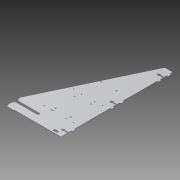
# Autodesk Inventor part: side_frame
Saved by Autodesk Inventor 2013 (Build 170138000, 138)
## iProperties
Created: 2013-11-17
Part Number: side_frame
Material: Generic
Document SubType Name: Modeling
Designer: Masta
Density: 1 g/cm^3
Author: Masta
Autodesk Inventor part; units mm, degrees
ref_plane "YZ Plane" through (0, 0, 0) normal (1, 0, 0) x (0, 1, 0)
ref_plane "XZ Plane" through (0, 0, 0) normal (0, 1, 0) x (-1, 0, 0)
ref_plane "XY Plane" through (0, 0, 0) normal (0, 0, 1) x (1, 0, 0)
sketch "Sketch1" plane through (0, 0, 0) normal (0, 0, 1) x (1, 0, 0)
  line L0 (255.7808, 350.0828) -> (255.7808, 358.8828)
  line L1 (251.6808, 67.29) -> (255.7808, 67.29)
  line L2 (255.7808, 67.29) -> (255.7808, 76.09)
  line L3 (255.7808, 76.09) -> (251.6808, 76.09)
  line L4 (251.6808, 76.09) -> (251.6808, 194.9901)
  line L5 (251.6808, 32.5401) -> (100.8808, 32.5401)
  line L6 (231.7439, 44.5401) -> (223.7479, 44.5401)
  line L7 (230.5808, 213.3401) -> (234.5808, 213.3401)
  line L8 (234.5808, 211.5401) -> (239.6808, 211.5401)
  line L9 (251.6808, 57.7345) -> (239.6808, 57.7345)
  line L10 (239.6808, 57.7345) -> (239.6808, 59.5345)
  line L11 (230.5808, 53.3345) -> (234.5808, 53.3345)
  line L12 (234.5808, 51.5345) -> (239.6808, 51.5345)
  line L13 (239.6808, 59.5345) -> (234.5808, 59.5345)
  line L14 (234.5808, 53.3345) -> (234.5808, 51.5345)
  line L15 (239.6808, 53.3345) -> (251.6808, 53.3345)
  line L16 (239.6808, 51.5345) -> (239.6808, 53.3345)
  line L17 (251.6808, 57.7345) -> (251.6808, 67.29)
  line L18 (251.6808, 217.7401) -> (239.6808, 217.7401)
  line L19 (255.7808, 236.0901) -> (251.6808, 236.0901)
  line L20 (251.6808, 236.0901) -> (251.6808, 350.0828)
  line L21 (255.7808, 203.7901) -> (251.6808, 203.7901)
  line L22 (251.6808, 194.9901) -> (255.7808, 194.9901)
  line L23 (255.7808, 194.9901) -> (255.7808, 203.7901)
  line L24 (251.6808, 227.2901) -> (251.6808, 217.7401)
  line L25 (251.6808, 213.3401) -> (251.6808, 203.7901)
  line L26 (251.6808, 382.3828) -> (255.7808, 382.3828)
  line L27 (255.7808, 382.3828) -> (255.7808, 391.1828)
  line L28 (255.7808, 391.1828) -> (251.6808, 391.1828)
  line L29 (251.6808, 391.1828) -> (251.6808, 400.5401)
  line L30 (255.7808, 358.8828) -> (251.6808, 358.8828)
  line L31 (251.6808, 350.0828) -> (255.7808, 350.0828)
  line L32 (73.8808, 35.5401) -> (73.8808, 51.1401)
  line L33 (239.6808, 211.5401) -> (239.6808, 213.3401)
  line L34 (230.5808, 217.7401) -> (230.5808, 213.3401)
  line L35 (73.8808, 77.5401) -> (226.2808, 400.5401)
  line L36 (234.5808, 217.7401) -> (230.5808, 217.7401)
  line L37 (234.5808, 217.7401) -> (234.5808, 219.5401)
  line L38 (251.6808, 400.5401) -> (226.2808, 400.5401)
  line L39 (239.6808, 213.3401) -> (251.6808, 213.3401)
  line L40 (231.7439, 36.5395) -> (223.7482, 36.5395)
  line L41 (239.6808, 219.5401) -> (234.5808, 219.5401)
  line L42 (98.8808, 30.5401) -> (78.8808, 30.5401)
  line L43 (234.5808, 213.3401) -> (234.5808, 211.5401)
  line L44 (230.5808, 372.825) -> (230.5808, 368.425)
  line L45 (234.5808, 372.825) -> (230.5808, 372.825)
  line L46 (234.5808, 372.825) -> (234.5808, 374.625)
  line L47 (251.6808, 372.825) -> (239.6808, 372.825)
  line L48 (230.5808, 368.425) -> (234.5808, 368.425)
  line L49 (239.6808, 368.425) -> (251.6808, 368.425)
  line L50 (234.5808, 366.625) -> (239.6808, 366.625)
  line L51 (239.6808, 374.625) -> (234.5808, 374.625)
  line L52 (234.5808, 368.425) -> (234.5808, 366.625)
  line L53 (251.6808, 372.825) -> (251.6808, 382.3828)
  line L54 (251.6808, 368.425) -> (251.6808, 358.8828)
  line L55 (230.5808, 57.7345) -> (230.5808, 53.3345)
  line L56 (234.5808, 57.7345) -> (230.5808, 57.7345)
  line L57 (234.5808, 57.7345) -> (234.5808, 59.5345)
  line L58 (239.6808, 366.625) -> (239.6808, 368.425)
  line L59 (239.6808, 372.825) -> (239.6808, 374.625)
  line L60 (78.8808, 56.1401) -> (148.8808, 56.1401)
  line L61 (78.8808, 56.1401) -> (73.8808, 51.1401)
  line L62 (78.8808, 64.9401) -> (148.8808, 64.9401)
  line L63 (73.8808, 69.9401) -> (73.8808, 77.5401)
  line L64 (78.8808, 64.9401) -> (73.8808, 69.9401)
  line L65 (251.6808, 227.2901) -> (255.7808, 227.2901)
  line L66 (255.7808, 227.2901) -> (255.7808, 236.0901)
  line L67 (239.6808, 217.7401) -> (239.6808, 219.5401)
  line L68 (78.8808, 30.5401) -> (73.8808, 35.5401)
  line L69 (100.8808, 32.5401) -> (98.8808, 30.5401)
  line L70 (251.6808, 32.5401) -> (251.6808, 53.3345)
  line L71 (136.6808, 189.5401) -> (231.6808, 189.5401) construction
  line L72 (231.6808, 189.5401) -> (231.6808, 93.5401) construction
  line L73 (231.6808, 93.5401) -> (136.6808, 93.5401) construction
  line L74 (136.6808, 93.5401) -> (136.6808, 189.5401) construction
  line L75 (164.6808, 93.5401) -> (208.6808, 93.5401) construction
  line L76 (208.6808, 93.5401) -> (208.6808, 187.5401) construction
  line L77 (208.6808, 187.5401) -> (164.6808, 187.5401) construction
  line L78 (164.6808, 187.5401) -> (164.6808, 93.5401) construction
  line L79 (160.3808, 93.5401) -> (208.6808, 93.5401) construction
  line L80 (208.6808, 93.5401) -> (208.6808, 168.5401) construction
  line L81 (208.6808, 168.5401) -> (160.3808, 168.5401) construction
  line L82 (160.3808, 168.5401) -> (160.3808, 93.5401) construction
  line L83 (208.6808, 168.5401) -> (208.6808, 174.8401) construction
  arc A0 (148.8808, 56.1401) -> (148.8808, 64.9401) centre (148.8808, 60.5401) ccw
  arc A1 (231.7439, 36.5395) -> (231.7439, 44.5401) centre (231.7439, 40.5398) ccw
  arc A2 (223.7479, 44.5401) -> (223.7482, 36.5395) centre (223.7482, 40.5398) ccw
  point P0 (0, 0)
  point P1 (219.7479, 40.5401)
  dimension "d0" = 177.8
  dimension "d9" = 95
  dimension "d10" = 96
  dimension "d11" = 44
  dimension "d12" = 94
  dimension "d15" = 48.3
  dimension "d16" = 75
  dimension "d18" = 6.3
  dimension "d19" = 23
  dimension "d20" = 20
  dimension "d21" = 63
  dimension "d22" = 4.1
  dimension "d23" = 8.8
  dimension "d46" = 8
  constraints: 168 end point, 17 collinear, 11 coincident, 7 parallel, 7 point on circle, 5 tangent, 4 horizontal, 3 centre point, 3 perpendicular, 1 vertical
  measures "d0" distance between parallel lines of L32 L70
  measures "d9" distance of L72.end L73.end
  measures "d10" distance of L71.end L72.end
  measures "d11" distance of L77.end L76.end
  measures "d12" distance of L75.end L76.end
  measures "d15" distance of L81.end L80.end
  measures "d16" distance of L80.end L75.end
  measures "d18" distance of L80.end L83.end
  measures "d19" distance between parallel lines of L72 L80
  measures "d20" distance between parallel lines of L4 L72
  measures "d21" distance between parallel lines of L42 L73
  measures "d22" distance between parallel lines of L2 L17
  measures "d23" distance of L1.end L2.end
  measures "d46" distance between parallel lines of L12 L13
extrude "Extrusion1" add sketch "Sketch1" against normal blind 4
hole "Hole1" at (136.6808, 189.5401, 0) at (136.6808, 93.5401, 0) at (231.6808, 93.5401, 0) at (231.6808, 189.5401, 0) at (160.3808, 93.5401, 0) at (208.6808, 93.5401, 0) at (208.6808, 174.8401, 0) at (160.3808, 168.5401, 0) at (164.6808, 93.5401, 0) at (164.6808, 187.5401, 0) at (208.6808, 187.5401, 0) direction (0, 0, -1) diameter 3.6 end through all
sketch "Sketch2" plane through (0, 0, 0) normal (0, 0, 1) x (1, 0, 0)
  line L0 (78.8808, 64.9401) -> (148.8808, 64.9401) projected
  line L1 (251.6808, 76.09) -> (251.6808, 194.9901) projected
  line L2 (162.1808, 104.9401) -> (212.1808, 104.9401) construction
  line L3 (212.1808, 104.9401) -> (212.1808, 254.9401) construction
  line L4 (212.1808, 254.9401) -> (162.1808, 254.9401) construction
  line L5 (162.1808, 254.9401) -> (162.1808, 104.9401) construction
  line L6 (162.1808, 104.9401) -> (212.1808, 254.9401) construction
  line L7 (212.1808, 104.9401) -> (162.1808, 254.9401) construction
  line L8 (129.6808, 69.9401) -> (244.6808, 69.9401) construction
  line L9 (244.6808, 69.9401) -> (244.6808, 289.9401) construction
  line L10 (244.6808, 289.9401) -> (129.6808, 289.9401) construction
  line L11 (129.6808, 289.9401) -> (129.6808, 69.9401) construction
  line L12 (129.6808, 69.9401) -> (244.6808, 289.9401) construction
  line L13 (244.6808, 69.9401) -> (129.6808, 289.9401) construction
  point P0 (0, 0)
  point P1 (187.1808, 179.9401)
  point P2 (187.1808, 179.9401)
  dimension "d33" = 50
  dimension "d34" = 150
  dimension "d35" = 115
  dimension "d36" = 220
  dimension "d37" = 5
  dimension "d38" = 7
  constraints: 24 end point, 5 midpoint, 4 coincident, 4 parallel, 2 horizontal, 2 perpendicular
  measures "d33" distance of L4.end L3.end
  measures "d34" distance of L3.end L2.end
  measures "d35" distance of L10.end L9.end
  measures "d36" distance of L9.end L8.end
  measures "d37" distance between parallel lines of L8 L0
  measures "d38" distance between parallel lines of L1 L9
hole "Hole2" at (162.1808, 254.9401, 0) at (162.1808, 104.9401, 0) at (212.1808, 104.9401, 0) at (212.1808, 254.9401, 0) direction (0, 0, -1) diameter 4.6 end through all
body "Solid1"
